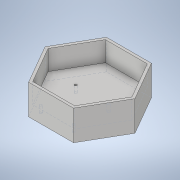
# Autodesk Inventor part: Internal Base
Saved by Autodesk Inventor 2020.2 (Build 242310000, 310)
## iProperties
Created: 2020-01-19
Part Number: Internal Base
Material: Generic
Document SubType Name: Modeling
Designer: prana
Density: 1 g/cm^3
Appearance: Default
Author: prana
Autodesk Inventor part; units mm, degrees
ref_plane "YZ Plane" through (0, 0, 0) normal (1, 0, 0) x (0, 1, 0)
ref_plane "XZ Plane" through (0, 0, 0) normal (0, 1, 0) x (-1, 0, 0)
ref_plane "XY Plane" through (0, 0, 0) normal (0, 0, 1) x (1, 0, 0)
sketch "Sketch1" plane through (0, 0, 0) normal (0, 1, 0) x (-1, 0, 0)
  line L0 (57.15, 0) -> (28.575, 49.4934)
  line L1 (28.575, 49.4934) -> (-28.575, 49.4934)
  line L2 (-28.575, 49.4934) -> (-57.15, 0)
  line L3 (57.15, 0) -> (28.575, -49.4934)
  line L4 (28.575, -49.4934) -> (-28.575, -49.4934)
  line L5 (-28.575, -49.4934) -> (-57.15, 0)
  point P0 (0, 0)
  dimension "d0" = 57.15
  dimension "d1" = 57.15
  dimension "d2" = 57.15
  dimension "d3" = 57.15
  constraints: 12 end point
  measures "d0" distance of point (0, 0) L0.start
  measures "d1" distance of L0.start L0.end
  measures "d2" distance of L0.end L1.end
  measures "d3" distance of L1.end L2.end
extrude "Extrusion1" add sketch "Sketch1" along normal blind 38.1
sketch "Sketch2" plane through (0, 38.1, 0) normal (0, 1, 0) x (1, 0, 0)
  line L0 (0, 0) -> (-53.34, 0)
  line L1 (-53.34, 0) -> (-26.67, -46.1938)
  line L2 (-26.67, -46.1938) -> (26.67, -46.1938)
  line L3 (26.67, -46.1938) -> (53.34, 0)
  line L4 (53.34, 0) -> (26.67, 46.1938)
  line L5 (26.67, 46.1938) -> (-26.67, 46.1938)
  line L6 (-26.67, 46.1938) -> (-53.34, 0)
  dimension "d6" = 53.34
  dimension "d7" = 53.34
  dimension "d8" = 60
  dimension "d9" = 53.34
  dimension "d10" = 53.34
  constraints: 14 end point, 4 parallel, 1 horizontal, 1 point on line
  measures "d6" distance of L0.start L0.end
  measures "d7" distance of L0.end L1.end
  measures "d8" angle of L1 L0
  measures "d9" distance of L1.end L2.end
  measures "d10" distance of L2.end L3.end
extrude "Extrusion2" cut sketch "Sketch2" against normal blind 31.75
sketch "Sketch3" plane through (0, 6.35, 0) normal (0, 1, 0) x (1, 0, 0)
  line L0 (26.67, -46.1938) -> (-26.67, -46.1938) projected
  line L1 (-26.67, -46.1938) -> (26.67, -46.1938)
  line L2 (53.34, 0) -> (26.67, -46.1938) projected
  line L3 (26.67, -46.1938) -> (53.34, 0)
  line L4 (-26.67, 46.1938) -> (26.67, 46.1938) projected
  line L5 (53.34, 0) -> (26.67, 46.1938)
  line L6 (26.67, 46.1938) -> (-26.67, 46.1938)
  line L7 (-26.67, 46.1938) -> (-53.34, 0)
  line L8 (-26.67, -46.1938) -> (-53.34, 0) projected
  line L9 (-53.34, 0) -> (-26.67, -46.1938)
  line L10 (-26.67, -46.1938) -> (26.67, -46.1938)
  point P0 (0, 0)
  constraints: 14 end point, 4 equal length, 1 horizontal
extrude "Extrusion3" add sketch "Sketch3" along normal blind 6.35
sketch "Sketch4" plane through (0, 12.7, 0) normal (0, 1, 0) x (1, 0, 0)
  circle A0 centre (-20.955, -41.7438) radius 1.5
  line L0 (26.67, -46.1938) -> (-26.67, -46.1938) projected
  circle A1 centre (20.955, -41.7438) radius 1.5
  circle A2 centre (-20.955, 2.7412) radius 1.5
  circle A3 centre (20.955, 2.7412) radius 1.5
  point P0 (0, 0)
  dimension "d15" = 3
  dimension "d16" = 4.45
  dimension "d17" = 3
  dimension "d18" = 41.91
  dimension "d19" = 20.955
  dimension "d20" = 4.45
  dimension "d21" = 3
  dimension "d22" = 44.485
  dimension "d23" = 20.955
  dimension "d24" = 3
  dimension "d25" = 41.91
  dimension "d26" = 44.485
  constraints: 4 centre point
  measures "d15" diameter of A0
  measures "d16" distance from line of L0 A0.centre
  measures "d17" diameter of A1
  measures "d18" distance of A1.centre A0.centre
  measures "d19" horizontal distance of point (0, 0) A0.centre
  measures "d20" distance from line of L0 A1.centre
  measures "d21" diameter of A2
  measures "d22" distance of A2.centre A0.centre
  measures "d23" horizontal distance of point (0, 0) A2.centre
  measures "d24" diameter of A3
  measures "d25" distance of A3.centre A2.centre
  measures "d26" distance of A1.centre A3.centre
extrude "Extrusion4" cut sketch "Sketch4" against normal blind 8.4667
body "Solid1"
